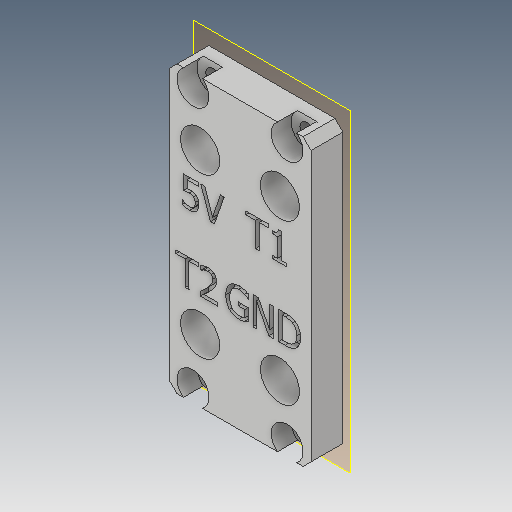
# Autodesk Inventor part: 02_Camera_Lid
Saved by Autodesk Inventor 2019 (Build 230136000, 136)
## iProperties
Created: 2021-09-23
Part Number: 02_Camera_Lid
Material: Generisch
Document SubType Name: Modeling
Designer: Muriel
Density: 1 g/cm^3
Appearance: Vorgabe
Author: Muriel
Autodesk Inventor part; units mm, degrees
ref_plane "YZ Plane" through (0, 0, 0) normal (1, 0, 0) x (0, 1, 0)
ref_plane "XZ Plane" through (0, 0, 0) normal (0, 1, 0) x (-1, 0, 0)
ref_plane "XY Plane" through (0, 0, 0) normal (0, 0, 1) x (1, 0, 0)
ref_plane "Arbeitsebene1" through (0, 0, 0) normal (0, 0, 1) x (1, 0, 0)
sketch "Skizze1" plane through (0, 0, 0) normal (0, 0, 1) x (1, 0, 0)
  line L0 (-3.05, 28.45) -> (-3.05, 27.95) projected
  line L1 (-2.75, 27.95) -> (-3.05, 27.95) projected
  line L2 (-1.75, 26.95) -> (-2.75, 27.95) projected
  line L3 (-1.75, 26.25) -> (-1.75, 26.95) projected
  line L4 (1.15, 26.25) -> (-1.75, 26.25) projected
  line L5 (1.15, 0.85) -> (1.15, 26.25) projected
  line L6 (1.15, 0.85) -> (-1.75, 0.85) projected
  line L7 (-1.75, 0.85) -> (-1.75, 0.15) projected
  line L8 (-2.75, -0.85) -> (-1.75, 0.15) projected
  line L9 (-2.75, -0.85) -> (-3.05, -0.85) projected
  line L10 (-3.05, -0.85) -> (-3.05, -1.35) projected
  line L11 (-3.05, -1.35) -> (-12.95, -1.35) projected
  line L12 (-12.95, -1.35) -> (-12.95, -0.35) projected
  line L13 (-12.95, -0.35) -> (-13.95, -0.35) projected
  line L14 (-13.95, -0.35) -> (-13.95, -1.35) projected
  line L15 (-13.95, -1.35) -> (-15.2198, -1.35) projected
  line L16 (-15.2198, -1.35) -> (-15.2198, 0.65) projected
  line L17 (-15.2198, 0.65) -> (-16.05, 0.65) projected
  line L18 (-16.05, 0.65) -> (-16.05, -3.35) projected
  line L19 (-15.05, -4.35) -> (-16.05, -3.35) projected
  line L20 (-15.05, -4.35) -> (0.75, -4.35) projected
  line L21 (1.75, -3.35) -> (0.75, -4.35) projected
  line L22 (1.75, -3.35) -> (1.75, 30.45) projected
  line L23 (0.75, 31.45) -> (1.75, 30.45) projected
  line L24 (-15.05, 31.45) -> (0.75, 31.45) projected
  line L25 (-16.05, 30.45) -> (-15.05, 31.45) projected
  line L26 (-16.05, 26.45) -> (-16.05, 30.45) projected
  line L27 (-16.05, 26.45) -> (-15.2198, 26.45) projected
  line L28 (-15.2198, 26.45) -> (-15.2198, 28.45) projected
  line L29 (-15.2198, 28.45) -> (-13.95, 28.45) projected
  line L30 (-13.95, 28.45) -> (-13.95, 27.45) projected
  line L31 (-13.95, 27.45) -> (-12.95, 27.45) projected
  line L32 (-12.95, 27.45) -> (-12.95, 28.45) projected
  line L33 (-12.95, 28.45) -> (-3.05, 28.45) projected
  circle A0 centre (-1.25, 29.85) radius 0.9 projected
  circle A1 centre (-13.05, 29.85) radius 0.9 projected
  circle A2 centre (-13.05, -2.75) radius 0.9 projected
  circle A3 centre (-1.25, -2.75) radius 0.9 projected
  line L34 (-16.05, 26.45) -> (-16.05, 0.65)
  point P0 (0, 0)
  constraints: 2 end point, 1 vertical
extrude "Extrusion1" add sketch "Skizze1" along normal blind 4
sketch "Skizze2" plane through (0, 0, 4) normal (0, 0, 1) x (1, 0, 0)
  circle A0 centre (-1.25, -2.75) radius 0.9 projected
  circle A1 centre (-13.05, -2.75) radius 0.9 projected
  circle A2 centre (-13.05, 29.85) radius 0.9 projected
  circle A3 centre (-1.25, 29.85) radius 0.9 projected
  line L0 (-16.05, 30.45) -> (-16.05, -3.35) projected
  line L1 (-16.05, -3.35) -> (-15.05, -4.35) projected
  line L2 (-15.05, -4.35) -> (0.75, -4.35) projected
  line L3 (0.75, -4.35) -> (1.75, -3.35) projected
  line L4 (1.75, -3.35) -> (1.75, 30.45) projected
  line L5 (1.75, 30.45) -> (0.75, 31.45) projected
  line L6 (0.75, 31.45) -> (-15.05, 31.45) projected
  line L7 (-15.05, 31.45) -> (-16.05, 30.45) projected
  point P0 (0, 0)
hole "Bohrung1" at (-1.25, 29.85, 4) at (-13.05, 29.85, 4) at (-1.25, -2.75, 4) at (-13.05, -2.75, 4) direction (0, 0, -1) diameter 1.8 depth 12 tip angle 118 counterbore diameter 4 counterbore depth 2.5
sketch "Skizze3" plane through (0, 0, 4) normal (0, 0, 1) x (1, 0, 0)
  arc A0 (-0.05, -4.35) -> (-2.45, -4.35) centre (-1.25, -2.75) ccw projected
  line L0 (-0.05, -4.35) -> (0.75, -4.35) projected
  line L1 (0.75, -4.35) -> (1.75, -3.35) projected
  line L2 (1.75, -3.35) -> (1.75, 30.45) projected
  line L3 (1.75, 30.45) -> (0.75, 31.45) projected
  line L4 (0.75, 31.45) -> (-0.05, 31.45) projected
  arc A1 (-2.45, 31.45) -> (-0.05, 31.45) centre (-1.25, 29.85) ccw projected
  line L5 (-2.45, 31.45) -> (-11.85, 31.45) projected
  arc A2 (-14.25, 31.45) -> (-11.85, 31.45) centre (-13.05, 29.85) ccw projected
  line L6 (-14.25, 31.45) -> (-15.05, 31.45) projected
  line L7 (-15.05, 31.45) -> (-16.05, 30.45) projected
  line L8 (-16.05, 30.45) -> (-16.05, -3.35) projected
  line L9 (-16.05, -3.35) -> (-15.05, -4.35) projected
  line L10 (-15.05, -4.35) -> (-14.25, -4.35) projected
  arc A3 (-11.85, -4.35) -> (-14.25, -4.35) centre (-13.05, -2.75) ccw projected
  line L11 (-11.85, -4.35) -> (-2.45, -4.35) projected
  line L12 (-12.15, 3.55) -> (-2.15, 3.55)
  line L13 (-2.15, 3.55) -> (-2.15, 23.55)
  line L14 (-2.15, 23.55) -> (-12.15, 23.55)
  line L15 (-12.15, 23.55) -> (-12.15, 3.55)
  line L16 (-12.15, 3.55) -> (-2.15, 23.55) construction
  line L17 (-2.15, 3.55) -> (-12.15, 23.55) construction
  circle A4 centre (-2.15, 23.55) radius 2.45
  circle A5 centre (-2.15, 3.55) radius 2.45
  circle A6 centre (-12.15, 3.55) radius 2.45
  circle A7 centre (-12.15, 23.55) radius 2.45
  point P0 (0, 0)
  point P1 (-7.15, 13.55)
  dimension "d9" = 10
  dimension "d10" = 20
  dimension "d11" = 4.9
  dimension "d12" = 4.9
  dimension "d13" = 4.9
  dimension "d14" = 4.9
  dimension "d15" = 17.8
  dimension "d16" = 8.9
  dimension "d17" = 35.8
  dimension "d18" = 17.9
  constraints: 12 end point, 4 centre point, 4 coincident, 2 midpoint, 2 parallel, 1 horizontal, 1 perpendicular
  measures "d9" distance of L14.end L13.end
  measures "d10" distance of L13.end L12.end
  measures "d11" diameter of A4
  measures "d12" diameter of A5
  measures "d13" diameter of A6
  measures "d14" diameter of A7
  measures "d15" distance between parallel lines of L8 L2
  measures "d16" distance from line of point (-7.15, 13.55) L2
  measures "d17" distance between parallel lines of L5 L11
  measures "d18" distance from line of L5 point (-7.15, 13.55)
extrude "Extrusion2" cut sketch "Skizze3" against normal blind 3.5 contours L15 A6 L12 | L12 A6 L15 | A5 L13 L12 | L12 L13 A5 | A7 L14 L15 | L15 L14 A7 | A4 L14 L13 | L13 L14 A4
sketch "Skizze4" plane through (0, 0, 4) normal (0, 0, 1) x (1, 0, 0)
  circle A0 centre (-12.15, 23.55) radius 2.45 projected
  circle A1 centre (-2.15, 3.55) radius 2.45 projected
  circle A2 centre (-2.15, 23.55) radius 2.45 projected
  circle A3 centre (-12.15, 3.55) radius 2.45 projected
  arc A4 (-0.05, -4.35) -> (-2.45, -4.35) centre (-1.25, -2.75) ccw projected
  line L0 (-0.05, -4.35) -> (0.75, -4.35) projected
  line L1 (0.75, -4.35) -> (1.75, -3.35) projected
  line L2 (1.75, -3.35) -> (1.75, 30.45) projected
  line L3 (1.75, 30.45) -> (0.75, 31.45) projected
  line L4 (0.75, 31.45) -> (-0.05, 31.45) projected
  arc A5 (-2.45, 31.45) -> (-0.05, 31.45) centre (-1.25, 29.85) ccw projected
  line L5 (-2.45, 31.45) -> (-11.85, 31.45) projected
  arc A6 (-14.25, 31.45) -> (-11.85, 31.45) centre (-13.05, 29.85) ccw projected
  line L6 (-14.25, 31.45) -> (-15.05, 31.45) projected
  line L7 (-15.05, 31.45) -> (-16.05, 30.45) projected
  line L8 (-16.05, 30.45) -> (-16.05, -3.35) projected
  line L9 (-16.05, -3.35) -> (-15.05, -4.35) projected
  line L10 (-15.05, -4.35) -> (-14.25, -4.35) projected
  arc A7 (-11.85, -4.35) -> (-14.25, -4.35) centre (-13.05, -2.75) ccw projected
  line L11 (-11.85, -4.35) -> (-2.45, -4.35) projected
  point P0 (0, 0)
hole "Bohrung2" at (-12.15, 23.55, 4) at (-2.15, 23.55, 4) at (-2.15, 3.55, 4) at (-12.15, 3.55, 4) direction (0, 0, -1) diameter 1 depth 12 tip angle 118
sketch "Skizze5" plane through (0, 0, 4) normal (0, 0, 1) x (1, 0, 0)
  line L0 (-14.6758, 19.919) -> (-9.1365, 19.919) construction
  line L1 (-9.1365, 19.919) -> (-9.1365, 16.3453) construction
  line L2 (-9.1365, 16.3453) -> (-14.6758, 16.3453) construction
  line L3 (-14.6758, 16.3453) -> (-14.6758, 19.919) construction
  line L4 (-9.0877, 11.2435) -> (0.5466, 11.2435) construction
  line L5 (0.5466, 11.2435) -> (0.5466, 7.613) construction
  line L6 (0.5466, 7.613) -> (-9.0877, 7.613) construction
  line L7 (-9.0877, 7.613) -> (-9.0877, 11.2435) construction
  line L8 (-6.4025, 19.8136) -> (-0.9653, 19.8136) construction
  line L9 (-0.9653, 19.8136) -> (-0.9653, 16.3023) construction
  line L10 (-0.9653, 16.3023) -> (-6.4025, 16.3023) construction
  line L11 (-6.4025, 16.3023) -> (-6.4025, 19.8136) construction
  line L12 (-15.191, 11.2782) -> (-9.7538, 11.2782) construction
  line L13 (-9.7538, 11.2782) -> (-9.7538, 7.7045) construction
  line L14 (-9.7538, 7.7045) -> (-15.191, 7.7045) construction
  line L15 (-15.191, 7.7045) -> (-15.191, 11.2782) construction
  spline S0 degree 2 poles (-12.299, 17.5309) (-12.299, 17.2784) (-12.4606, 16.8473) (-12.6081, 16.6885) knots 0 0 0 1 2 2 2
  spline S1 degree 2 poles (-12.6081, 16.6885) (-12.7556, 16.5296) (-13.1952, 16.3453) (-13.4675, 16.3453) knots 0 0 0 1 2 2 2
  spline S2 degree 2 poles (-13.4675, 16.3453) (-13.7171, 16.3453) (-14.205, 16.4559) (-14.3837, 16.5438) knots 0 0 0 1 2 2 2
  line L16 (-14.3837, 16.5438) -> (-14.3837, 17.0402)
  line L17 (-14.3837, 17.0402) -> (-14.3496, 17.0402)
  spline S3 degree 2 poles (-14.3496, 17.0402) (-14.2957, 17.0005) (-14.0943, 16.8984) (-13.9724, 16.853) knots 0 0 0 1 2 2 2
  spline S4 degree 2 poles (-13.9724, 16.853) (-13.8334, 16.8048) (-13.6037, 16.7509) (-13.459, 16.7509) knots 0 0 0 1 2 2 2
  spline S5 degree 2 poles (-13.459, 16.7509) (-13.3172, 16.7509) (-13.0506, 16.853) (-12.9542, 16.9636) knots 0 0 0 1 2 2 2
  spline S6 degree 2 poles (-12.9542, 16.9636) (-12.8662, 17.0685) (-12.7755, 17.3465) (-12.7755, 17.5337) knots 0 0 0 1 2 2 2
  spline S7 degree 2 poles (-12.7755, 17.5337) (-12.7755, 17.7209) (-12.8776, 17.9591) (-12.974, 18.0386) knots 0 0 0 1 2 2 2
  spline S8 degree 2 poles (-12.974, 18.0386) (-13.0733, 18.1265) (-13.3683, 18.2002) (-13.5469, 18.2002) knots 0 0 0 1 2 2 2
  spline S9 degree 2 poles (-13.5469, 18.2002) (-13.7398, 18.2002) (-14.1227, 18.1407) (-14.239, 18.1151) knots 0 0 0 1 2 2 2
  line L18 (-14.239, 18.1151) -> (-14.239, 19.919)
  line L19 (-14.239, 19.919) -> (-12.3188, 19.919)
  line L20 (-12.3188, 19.919) -> (-12.3188, 19.5078)
  line L21 (-12.3188, 19.5078) -> (-13.788, 19.5078)
  line L22 (-13.788, 19.5078) -> (-13.788, 18.5746)
  spline S10 degree 2 poles (-13.788, 18.5746) (-13.7029, 18.586) (-13.5384, 18.5945) (-13.4704, 18.5945) knots 0 0 0 1 2 2 2
  spline S11 degree 2 poles (-13.4704, 18.5945) (-13.2009, 18.5945) (-12.8294, 18.5065) (-12.6592, 18.3761) knots 0 0 0 1 2 2 2
  spline S12 degree 2 poles (-12.6592, 18.3761) (-12.4862, 18.2456) (-12.299, 17.8485) (-12.299, 17.5309) knots 0 0 0 1 2 2 2
  line L23 (-9.1563, 19.919) -> (-10.3618, 16.419)
  line L24 (-10.3618, 16.419) -> (-10.8638, 16.419)
  line L25 (-10.8638, 16.419) -> (-12.0692, 19.919)
  line L26 (-12.0692, 19.919) -> (-11.57, 19.919)
  line L27 (-11.57, 19.919) -> (-10.6, 17.0118)
  line L28 (-10.6, 17.0118) -> (-9.63, 19.919)
  line L29 (-9.63, 19.919) -> (-9.1563, 19.919)
  line L30 (-5.2311, 16.3023) -> (-5.2311, 19.3882)
  line L31 (-5.2311, 19.3882) -> (-6.4054, 19.3882)
  line L32 (-6.4054, 19.3882) -> (-6.4054, 19.8023)
  line L33 (-6.4054, 19.8023) -> (-3.5918, 19.8023)
  line L34 (-3.5918, 19.8023) -> (-3.5918, 19.3882)
  line L35 (-3.5918, 19.3882) -> (-4.766, 19.3882)
  line L36 (-4.766, 19.3882) -> (-4.766, 16.3023)
  line L37 (-4.766, 16.3023) -> (-5.2311, 16.3023)
  line L38 (-1.3539, 16.3023) -> (-3.0614, 16.3023)
  line L39 (-3.0614, 16.3023) -> (-3.0614, 16.6597)
  line L40 (-3.0614, 16.6597) -> (-2.426, 16.6597)
  line L41 (-2.426, 16.6597) -> (-2.426, 19.0053)
  line L42 (-2.426, 19.0053) -> (-3.0614, 19.0053)
  line L43 (-3.0614, 19.0053) -> (-3.0614, 19.3258)
  spline S13 degree 2 poles (-3.0614, 19.3258) (-2.7012, 19.3258) (-2.3608, 19.53) (-2.3381, 19.8136) knots 0 0 0 1 2 2 2
  line L44 (-2.3381, 19.8136) -> (-1.9751, 19.8136)
  line L45 (-1.9751, 19.8136) -> (-1.9751, 16.6597)
  line L46 (-1.9751, 16.6597) -> (-1.3539, 16.6597)
  line L47 (-1.3539, 16.6597) -> (-1.3539, 16.3023)
  spline S14 degree 2 poles (-7.2668, 7.613) (-7.6384, 7.613) (-8.2538, 7.8399) (-8.4751, 8.0696) knots 0 0 0 1 2 2 2
  spline S15 degree 2 poles (-8.4751, 8.0696) (-8.6963, 8.3022) (-8.9317, 8.9886) (-8.9317, 9.4339) knots 0 0 0 1 2 2 2
  spline S16 degree 2 poles (-8.9317, 9.4339) (-8.9317, 9.8565) (-8.6935, 10.5259) (-8.4722, 10.7641) knots 0 0 0 1 2 2 2
  spline S17 degree 2 poles (-8.4722, 10.7641) (-8.2595, 10.9939) (-7.6355, 11.2435) (-7.264, 11.2435) knots 0 0 0 1 2 2 2
  spline S18 degree 2 poles (-7.264, 11.2435) (-7.0853, 11.2435) (-6.7619, 11.1924) (-6.6144, 11.147) knots 0 0 0 1 2 2 2
  spline S19 degree 2 poles (-6.6144, 11.147) (-6.4953, 11.113) (-6.206, 10.9882) (-6.1181, 10.9428) knots 0 0 0 1 2 2 2
  line L48 (-6.1181, 10.9428) -> (-6.1181, 10.3812)
  line L49 (-6.1181, 10.3812) -> (-6.1578, 10.3812)
  spline S20 degree 2 poles (-6.1578, 10.3812) (-6.2457, 10.4578) (-6.4301, 10.5968) (-6.6003, 10.6762) knots 0 0 0 1 2 2 2
  spline S21 degree 2 poles (-6.6003, 10.6762) (-6.7421, 10.7471) (-7.108, 10.8407) (-7.3179, 10.8407) knots 0 0 0 1 2 2 2
  spline S22 degree 2 poles (-7.3179, 10.8407) (-7.8227, 10.8407) (-8.4467, 10.0806) (-8.4467, 9.4481) knots 0 0 0 1 2 2 2
  spline S23 degree 2 poles (-8.4467, 9.4481) (-8.4467, 9.0964) (-8.2822, 8.5688) (-8.1262, 8.3873) knots 0 0 0 1 2 2 2
  spline S24 degree 2 poles (-8.1262, 8.3873) (-7.9759, 8.2058) (-7.5504, 8.0157) (-7.2838, 8.0157) knots 0 0 0 1 2 2 2
  spline S25 degree 2 poles (-7.2838, 8.0157) (-7.0881, 8.0157) (-6.6967, 8.0725) (-6.5634, 8.1292) knots 0 0 0 1 2 2 2
  line L50 (-6.5634, 8.1292) -> (-6.5634, 9.034)
  line L51 (-6.5634, 9.034) -> (-7.3746, 9.034)
  line L52 (-7.3746, 9.034) -> (-7.3746, 9.4424)
  line L53 (-7.3746, 9.4424) -> (-6.1039, 9.4424)
  line L54 (-6.1039, 9.4424) -> (-6.1039, 7.9136)
  spline S26 degree 2 poles (-6.1039, 7.9136) (-6.1918, 7.8739) (-6.4925, 7.752) (-6.6201, 7.7151) knots 0 0 0 1 2 2 2
  spline S27 degree 2 poles (-6.6201, 7.7151) (-6.7931, 7.664) (-7.0711, 7.613) (-7.2668, 7.613) knots 0 0 0 1 2 2 2
  line L55 (-3.0152, 7.6811) -> (-3.5371, 7.6811)
  line L56 (-3.5371, 7.6811) -> (-5.0857, 10.6989)
  line L57 (-5.0857, 10.6989) -> (-5.0857, 7.6811)
  line L58 (-5.0857, 7.6811) -> (-5.5196, 7.6811)
  line L59 (-5.5196, 7.6811) -> (-5.5196, 11.1811)
  line L60 (-5.5196, 11.1811) -> (-4.8588, 11.1811)
  line L61 (-4.8588, 11.1811) -> (-3.4491, 8.41)
  line L62 (-3.4491, 8.41) -> (-3.4491, 11.1811)
  line L63 (-3.4491, 11.1811) -> (-3.0152, 11.1811)
  line L64 (-3.0152, 11.1811) -> (-3.0152, 7.6811)
  spline S28 degree 2 poles (0.4536, 9.4282) (0.4536, 8.9489) (0.065, 8.1774) (-0.2611, 7.9619) knots 0 0 0 1 2 2 2
  spline S29 degree 2 poles (-0.2611, 7.9619) (-0.5277, 7.7945) (-1.0751, 7.6811) (-1.5006, 7.6811) knots 0 0 0 1 2 2 2
  line L65 (-1.5006, 7.6811) -> (-2.3061, 7.6811)
  line L66 (-2.3061, 7.6811) -> (-2.3061, 11.1811)
  line L67 (-2.3061, 11.1811) -> (-1.5091, 11.1811)
  spline S30 degree 2 poles (-1.5091, 11.1811) (-1.0156, 11.1811) (-0.454, 11.0336) (-0.2555, 10.9031) knots 0 0 0 1 2 2 2
  spline S31 degree 2 poles (-0.2555, 10.9031) (0.0821, 10.679) (0.4536, 9.9388) (0.4536, 9.4282) knots 0 0 0 1 2 2 2
  spline S32 degree 2 poles (-0.0314, 9.4339) (-0.0314, 9.8367) (-0.298, 10.4068) (-0.5618, 10.5684) knots 0 0 0 1 2 2 2
  spline S33 degree 2 poles (-0.5618, 10.5684) (-0.749, 10.679) (-1.1716, 10.7783) (-1.4864, 10.7783) knots 0 0 0 1 2 2 2
  line L68 (-1.4864, 10.7783) -> (-1.8409, 10.7783)
  line L69 (-1.8409, 10.7783) -> (-1.8409, 8.0838)
  line L70 (-1.8409, 8.0838) -> (-1.4864, 8.0838)
  spline S34 degree 2 poles (-1.4864, 8.0838) (-1.1773, 8.0838) (-0.7093, 8.1831) (-0.5192, 8.3164) knots 0 0 0 1 2 2 2
  spline S35 degree 2 poles (-0.5192, 8.3164) (-0.2753, 8.4809) (-0.0314, 9.0255) (-0.0314, 9.4339) knots 0 0 0 1 2 2 2
  line L71 (-14.0196, 7.7045) -> (-14.0196, 10.7904)
  line L72 (-14.0196, 10.7904) -> (-15.1939, 10.7904)
  line L73 (-15.1939, 10.7904) -> (-15.1939, 11.2045)
  line L74 (-15.1939, 11.2045) -> (-12.3803, 11.2045)
  line L75 (-12.3803, 11.2045) -> (-12.3803, 10.7904)
  line L76 (-12.3803, 10.7904) -> (-13.5545, 10.7904)
  line L77 (-13.5545, 10.7904) -> (-13.5545, 7.7045)
  line L78 (-13.5545, 7.7045) -> (-14.0196, 7.7045)
  line L79 (-9.9666, 7.7045) -> (-12.125, 7.7045)
  line L80 (-12.125, 7.7045) -> (-12.125, 8.2009)
  spline S36 degree 2 poles (-12.125, 8.2009) (-11.8924, 8.4192) (-11.4783, 8.8248) (-11.2798, 9.0432) knots 0 0 0 1 2 2 2
  spline S37 degree 2 poles (-11.2798, 9.0432) (-10.8798, 9.4829) (-10.5877, 10.0104) (-10.5877, 10.2912) knots 0 0 0 1 2 2 2
  spline S38 degree 2 poles (-10.5877, 10.2912) (-10.5877, 10.4387) (-10.6785, 10.6599) (-10.7607, 10.7308) knots 0 0 0 1 2 2 2
  spline S39 degree 2 poles (-10.7607, 10.7308) (-10.843, 10.8017) (-11.0585, 10.8726) (-11.189, 10.8726) knots 0 0 0 1 2 2 2
  spline S40 degree 2 poles (-11.189, 10.8726) (-11.3138, 10.8726) (-11.5691, 10.8103) (-11.6854, 10.762) knots 0 0 0 1 2 2 2
  spline S41 degree 2 poles (-11.6854, 10.762) (-11.7846, 10.7223) (-11.969, 10.6089) (-12.0257, 10.5692) knots 0 0 0 1 2 2 2
  line L81 (-12.0257, 10.5692) -> (-12.0512, 10.5692)
  line L82 (-12.0512, 10.5692) -> (-12.0512, 11.0684)
  spline S42 degree 2 poles (-12.0512, 11.0684) (-11.9066, 11.1393) (-11.3875, 11.2782) (-11.155, 11.2782) knots 0 0 0 1 2 2 2
  spline S43 degree 2 poles (-11.155, 11.2782) (-10.6643, 11.2782) (-10.1112, 10.7592) (-10.1112, 10.3167) knots 0 0 0 1 2 2 2
  spline S44 degree 2 poles (-10.1112, 10.3167) (-10.1112, 10.1097) (-10.2076, 9.7637) (-10.2927, 9.6162) knots 0 0 0 1 2 2 2
  spline S45 degree 2 poles (-10.2927, 9.6162) (-10.3778, 9.463) (-10.6246, 9.1624) (-10.7607, 9.0177) knots 0 0 0 1 2 2 2
  spline S46 degree 2 poles (-10.7607, 9.0177) (-10.982, 8.7766) (-11.5237, 8.2604) (-11.6854, 8.1101) knots 0 0 0 1 2 2 2
  line L83 (-11.6854, 8.1101) -> (-9.9666, 8.1101)
  line L84 (-9.9666, 8.1101) -> (-9.9666, 7.7045)
  point P0 (0, 0)
  constraints: 8 other
extrude "Extrusion3" cut sketch "Skizze5" against normal blind 1
equation "\"d16\" = 0.5 * d15"
equation "\"d18\" = 0.5 * d17"
